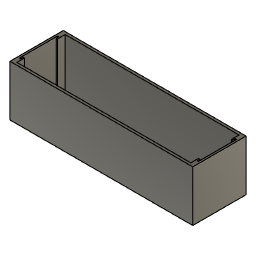
hbat (Autodesk Fusion 360 design; units mm, degrees)
Autodesk Fusion 360 part; units mm, degrees
sketch "Sketch1" plane through (0, 0, 0) normal (0, 0, 1) x (1, 0, 0)
  line L0 (0, 0) -> (72, 0)
  line L1 (72, 0) -> (72, 21)
  line L2 (72, 21) -> (0, 21)
  line L3 (0, 21) -> (0, 0)
  line L4 (4.75, 20) -> (69.75, 20)
  line L5 (69.75, 20) -> (69.75, 1)
  line L6 (69.75, 1) -> (4.75, 1)
  line L7 (4.75, 1) -> (4.75, 20)
  line L8 (69.75, 20) -> (71.25, 20)
  line L9 (71.25, 20) -> (71.25, 1)
  line L10 (71.25, 1) -> (69.75, 1)
  line L11 (69.75, 1) -> (69.75, 20)
  line L12 (4.75, 20) -> (0.75, 20)
  line L13 (0.75, 20) -> (0.75, 1)
  line L14 (0.75, 1) -> (4.75, 1)
  line L15 (4.75, 1) -> (4.75, 20)
  line L16 (0.75, 18) -> (1.25, 18)
  line L17 (1.25, 18) -> (1.25, 3)
  line L18 (1.25, 3) -> (0.75, 3)
  line L19 (0.75, 3) -> (0.75, 18)
  line L20 (1.25, 14.5) -> (4.75, 14.5)
  line L21 (4.75, 14.5) -> (4.75, 6.5)
  line L22 (4.75, 6.5) -> (1.25, 6.5)
  line L23 (1.25, 6.5) -> (1.25, 14.5)
  line L24 (0.75, 20) -> (1.75, 20)
  line L25 (1.75, 20) -> (1.75, 18)
  line L26 (1.75, 18) -> (0.75, 18)
  line L27 (0.75, 18) -> (0.75, 20)
  line L28 (1.75, 18) -> (1.25, 18)
  line L29 (1.25, 18) -> (1.25, 17)
  line L30 (1.25, 17) -> (1.75, 17)
  line L31 (1.75, 17) -> (1.75, 18)
  line L32 (0.75, 3) -> (1.75, 3)
  line L33 (1.75, 3) -> (1.75, 1)
  line L34 (1.75, 1) -> (0.75, 1)
  line L35 (0.75, 1) -> (0.75, 3)
  line L36 (1.25, 3) -> (1.75, 3)
  line L37 (1.75, 3) -> (1.75, 4)
  line L38 (1.75, 4) -> (1.25, 4)
  line L39 (1.25, 4) -> (1.25, 3)
  line L40 (71.25, 18) -> (70.75, 18)
  line L41 (70.75, 18) -> (70.75, 3)
  line L42 (70.75, 3) -> (71.25, 3)
  line L43 (71.25, 3) -> (71.25, 18)
  line L44 (70.75, 14.5) -> (69.75, 14.5)
  line L45 (69.75, 14.5) -> (69.75, 6.5)
  line L46 (69.75, 6.5) -> (70.75, 6.5)
  line L47 (70.75, 6.5) -> (70.75, 14.5)
  line L48 (71.25, 20) -> (70.25, 20)
  line L49 (70.25, 20) -> (70.25, 18)
  line L50 (70.25, 18) -> (71.25, 18)
  line L51 (71.25, 18) -> (71.25, 20)
  line L52 (70.25, 18) -> (70.75, 18)
  line L53 (70.75, 18) -> (70.75, 17)
  line L54 (70.75, 17) -> (70.25, 17)
  line L55 (70.25, 17) -> (70.25, 18)
  line L56 (71.25, 3) -> (70.25, 3)
  line L57 (70.25, 3) -> (70.25, 1)
  line L58 (70.25, 1) -> (71.25, 1)
  line L59 (71.25, 1) -> (71.25, 3)
  line L60 (70.25, 3) -> (70.75, 3)
  line L61 (70.75, 3) -> (70.75, 4)
  line L62 (70.75, 4) -> (70.25, 4)
  line L63 (70.25, 4) -> (70.25, 3)
  dimension "d46" = 72
  dimension "d47" = 21
  dimension "d48" = 65
  dimension "d49" = 19
  dimension "d50" = 1
  dimension "d51" = 1.5
  dimension "d52" = 19
  dimension "d53" = 4
  dimension "d54" = 19
  dimension "d55" = 0.75
  dimension "d56" = 0.5
  dimension "d57" = 15
  dimension "d58" = 2
  dimension "d59" = 8
  dimension "d60" = 3.5
  dimension "d61" = 3.5
  dimension "d62" = 1
  dimension "d63" = 2
  dimension "d64" = 0.5
  dimension "d65" = 1
  dimension "d66" = 1
  dimension "d67" = 2
  dimension "d68" = 0.5
  dimension "d69" = 1
  dimension "d70" = 0.5
  dimension "d71" = 15
  dimension "d72" = 2
  dimension "d73" = 1
  dimension "d74" = 8
  dimension "d75" = 3.5
  dimension "d76" = 1
  dimension "d77" = 2
  dimension "d78" = 0.5
  dimension "d79" = 1
  dimension "d80" = 1
  dimension "d81" = 2
  dimension "d82" = 0.5
  dimension "d83" = 1
  constraint horizontal L0
  constraint vertical L1
  constraint horizontal L2
  constraint vertical L3
  constraint coincident L0.start L3.end
  constraint horizontal L4
  constraint vertical L5
  constraint horizontal L6
  constraint vertical L7
  constraint horizontal L8
  constraint vertical L9
  constraint horizontal L10
  constraint vertical L11
  constraint horizontal L12
  constraint vertical L13
  constraint horizontal L14
  constraint vertical L15
  constraint horizontal L16
  constraint vertical L17
  constraint horizontal L18
  constraint vertical L19
  constraint coincident L13 L16.start
  constraint horizontal L20
  constraint vertical L21
  constraint horizontal L22
  constraint vertical L23
  constraint coincident L17 L20.start
  constraint horizontal L24
  constraint vertical L25
  constraint horizontal L26
  constraint vertical L27
  constraint horizontal L28
  constraint vertical L29
  constraint horizontal L30
  constraint vertical L31
  constraint horizontal L32
  constraint vertical L33
  constraint horizontal L34
  constraint vertical L35
  constraint horizontal L36
  constraint vertical L37
  constraint horizontal L38
  constraint vertical L39
  constraint horizontal L40
  constraint vertical L41
  constraint horizontal L42
  constraint vertical L43
  constraint coincident L9 L40.start
  constraint horizontal L44
  constraint vertical L45
  constraint horizontal L46
  constraint vertical L47
  constraint coincident L41 L44.start
  constraint horizontal L48
  constraint vertical L49
  constraint horizontal L50
  constraint vertical L51
  constraint horizontal L52
  constraint vertical L53
  constraint horizontal L54
  constraint vertical L55
  constraint horizontal L56
  constraint vertical L57
  constraint horizontal L58
  constraint vertical L59
  constraint horizontal L60
  constraint vertical L61
  constraint horizontal L62
  constraint vertical L63
  measures "d46" distance of L0.start L0.end
  measures "d47" distance of L0.start L2.end
  measures "d48" distance of L4.start L4.end
  measures "d49" distance of L4.start L6.end
  measures "d50" distance of L2 L4
  measures "d51" distance of L4.end L8.end
  measures "d52" distance of L4.end L5.end
  measures "d53" distance of L4.start L12.end
  measures "d54" distance of L4.start L6.end
  measures "d55" distance of L3 L13
  measures "d56" distance of L16.start L16.end
  measures "d57" distance of L16.start L18.end
  measures "d58" distance of L12 L16
  measures "d59" distance of L20.start L22.end
  measures "d60" distance of L16 L20
  measures "d61" distance of L20.start L20.end
  measures "d62" distance of L12.end L24.end
  measures "d63" distance of L12.end L16.start
  measures "d64" distance of L25.end L16.end
  measures "d65" distance of L25.end L30.end
  measures "d66" distance of L18.end L32.end
  measures "d67" distance of L18.end L13.end
  measures "d68" distance of L17.end L32.end
  measures "d69" distance of L17.end L38.end
  measures "d70" distance of L40.start L40.end
  measures "d71" distance of L40.start L42.end
  measures "d72" distance of L8 L40
  measures "d73" distance of L44.start L44.end
  measures "d74" distance of L44.start L46.end
  measures "d75" distance of L40 L44
  measures "d76" distance of L8.end L48.end
  measures "d77" distance of L8.end L40.start
  measures "d78" distance of L49.end L40.end
  measures "d79" distance of L49.end L54.end
  measures "d80" distance of L42.end L56.end
  measures "d81" distance of L42.end L9.end
  measures "d82" distance of L56.end L41.end
  measures "d83" distance of L56.end L62.end
extrude "Extrude3" add sketch "Sketch1" against normal blind 1 contours L0 L1 L2 L3 | L4 L5 L6 L7 L11 L15 L21 L45 | L7 L12 L15 L17 L20 L25 L30 L31 | L5 L8 L11 L41 L44 L49 L54 L55 | L7 L15 L17 L20 L21 L22 L23 | L12 L13 L16 L24 L25 L26 L27 L28 | L5 L11 L41 L44 L45 L46 L47 | L8 L9 L40 L48 L49 L50 L51 L52 | L7 L14 L15 L17 L22 L33 L37 L38 | L13 L16 L17 L18 L19 L23 L26 L29 L32 L39 | L17 L26 L28 L29 L30 L31 | L5 L10 L11 L41 L46 L57 L62 L63 | L9 L40 L41 L42 L43 L47 L50 L53 L56 L61 | L41 L50 L52 L53 L54 L55 | L13 L14 L18 L32 L33 L34 L35 L36 | L17 L32 L36 L37 L38 L39 | L9 L10 L42 L56 L57 L58 L59 L60 | L41 L56 L60 L61 L62 L63
extrude "Extrude4" add sketch "Sketch1" along normal blind 19 contours L0 L1 L2 L3 | L12 L13 L16 L24 L25 L26 L27 L28 | L8 L9 L40 L48 L49 L50 L51 L52 | L17 L26 L28 L29 L30 L31 | L41 L50 L52 L53 L54 L55 | L13 L14 L18 L32 L33 L34 L35 L36 | L17 L32 L36 L37 L38 L39 | L9 L10 L42 L56 L57 L58 L59 L60 | L41 L56 L60 L61 L62 L63
extrude "Extrude5" add sketch "Sketch1" along normal blind 3 contours L13 L16 L17 L18 L19 L23 L26 L29 L32 L39 | L9 L40 L41 L42 L43 L47 L50 L53 L56 L61
